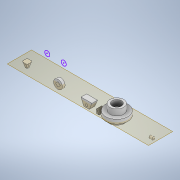
# Autodesk Inventor part: Lab1
Saved by Autodesk Inventor 2021.1 (Build 251245010, 245A)
## iProperties
Created: 2023-09-14
Part Number: Lab1
Material: Типовые
Document SubType Name: Modeling
Designer: Lenovo
Density: 1 g/cm^3
Appearance: По умолчанию
Author: Lenovo
Autodesk Inventor part; units mm, degrees
ref_plane "YZ Plane" through (0, 0, 0) normal (1, 0, 0) x (0, 1, 0)
ref_plane "XY Plane" through (0, 0, 0) normal (0, 0, 1) x (1, 0, 0)
sketch "Эскиз3" plane through (0, 0, 0) normal (0, 0, 1) x (1, 0, 0)
  line L0 (0, 0) -> (10, 0)
  line L1 (10, 0) -> (1.8715, 12.051)
  line L2 (1.8715, 12.051) -> (0, 14.8256)
  line L3 (0, 14.8256) -> (0, 0)
  dimension "d0" = 10
  dimension "d1" = 56
  constraints: 8 end point, 1 horizontal, 1 perpendicular, 1 point on line
  measures "d0" distance of L0.start L0.end
  measures "d1" angle of L1 L0
sketch "Эскиз4" plane through (0, 0, 0) normal (0, 0, 1) x (1, 0, 0)
  line L0 (-46.0484, 0) -> (-26.0484, 0)
  line L1 (-16.0484, 24) -> (-26.0484, 0)
  line L2 (-56.0484, 24) -> (-46.0484, 0)
  circle A0 centre (-36.0484, 8) radius 4
  line L3 (-36.0484, 24) -> (-56.0484, 24)
  line L4 (-36.0484, 24) -> (-16.0484, 24)
  point P0 (0, 0)
  dimension "d2" = 20
  dimension "d8" = 8
  dimension "d10" = 20
  dimension "d11" = 20
  dimension "d12" = 16
  constraints: 10 end point, 2 horizontal, 1 centre point
  measures "d2" distance of L0.start L0.end
  measures "d8" diameter of A0
  measures "d10" distance of L3.start L2.start
  measures "d11" distance of L3.start L1.start
  measures "d12" distance of L3.start A0.centre
sketch "Эскиз5" plane through (0, 0, 0) normal (0, 0, 1) x (1, 0, 0)
  line L0 (60.0217, 0) -> (66.0217, 0)
  line L1 (66.0217, 0) -> (66.0217, 8)
  line L2 (66.0217, 8) -> (74.0217, 8)
  line L3 (74.0217, 8) -> (74.0217, 0)
  line L4 (74.0217, 0) -> (82.0217, 0)
  line L5 (82.0217, 0) -> (82.0217, 12)
  line L6 (82.0217, 12) -> (94.0217, 12)
  line L7 (94.0217, 12) -> (94.0217, 27)
  line L8 (94.0217, 27) -> (79.0217, 27)
  line L9 (79.0217, 27) -> (79.0217, 49)
  line L10 (79.0217, 49) -> (71.0217, 49)
  line L11 (71.0217, 49) -> (71.0217, 29)
  line L12 (71.0217, 29) -> (60.0217, 29)
  line L13 (60.0217, 29) -> (60.0217, 0)
  line L14 (60.0217, 0) -> (54.0217, 0)
  line L15 (54.0217, 15.2415) -> (54.0217, -9.2055)
  point P0 (0, 0)
  dimension "d13" = 6
  dimension "d14" = 8
  dimension "d15" = 8
  dimension "d16" = 8
  dimension "d17" = 8
  dimension "d18" = 12
  dimension "d19" = 12
  dimension "d20" = 15
  dimension "d21" = 15
  dimension "d22" = 22
  dimension "d23" = 8
  dimension "d24" = 20
  dimension "d25" = 11
  dimension "d76" = 6
  constraints: 32 end point, 10 perpendicular, 2 horizontal, 2 point on line, 1 coincident, 1 vertical
  measures "d13" distance of L0.start L0.end
  measures "d14" distance of L0.end L1.end
  measures "d15" distance of L1.end L2.end
  measures "d16" distance of L2.end L3.end
  measures "d17" distance of L3.end L4.end
  measures "d18" distance of L4.end L5.end
  measures "d19" distance of L5.end L6.end
  measures "d20" distance of L6.end L7.end
  measures "d21" distance of L7.end L8.end
  measures "d22" distance of L8.end L9.end
  measures "d23" distance of L9.end L10.end
  measures "d24" distance of L10.end L11.end
  measures "d25" distance of L11.end L12.end
  measures "d76" distance of L0.start L14.end
sketch "Эскиз6" plane through (0, 0, 0) normal (0, 0, 1) x (1, 0, 0)
  circle A0 centre (-150.007, 11.9827) radius 16
  line L0 (-150.007, 20.468) -> (-141.5218, 11.9827)
  line L1 (-158.4923, 11.9827) -> (-150.007, 3.4975)
  line L2 (-150.007, 3.4975) -> (-141.5218, 11.9827)
  line L3 (-141.5218, 11.9827) -> (-150.007, 3.4975)
  line L4 (-158.4923, 11.9827) -> (-150.007, 20.468)
  point P0 (0, 0)
  constraints: 10 end point, 3 perpendicular, 1 centre point
sketch "Эскиз7" plane through (0, 0, 0) normal (0, 0, 1) x (1, 0, 0)
  point P0 (0, 0)
sketch "Эскиз8" plane through (0, 0, 0) normal (0, 0, 1) x (1, 0, 0)
  line L0 (175.9744, 1.9848) -> (175.9744, -0.0152)
  line L1 (175.9744, -0.0152) -> (186.7744, -0.0152)
  line L2 (175.9744, 1.9848) -> (186.7744, 1.9848)
  line L3 (186.7744, 1.9848) -> (186.7744, 1.9848)
  line L4 (187.9744, 3.1848) -> (187.9744, 3.1848)
  line L5 (189.9744, 3.1848) -> (189.9744, 3.1848)
  line L6 (186.7744, -0.0152) -> (186.7744, -0.0152)
  line L7 (186.7744, -0.0152) -> (186.7744, -0.0152)
  line L8 (189.9744, 3.1848) -> (189.9744, 3.4848)
  line L9 (189.9744, 3.4848) -> (187.9744, 3.4848)
  line L10 (187.9744, 3.4848) -> (187.9744, 3.1848)
  line L11 (186.7744, 1.9848) -> (186.7744, 1.9848)
  arc A0 (186.7744, -0.0152) -> (189.9744, 3.1848) centre (186.7744, 3.1848) ccw
  arc A1 (186.7744, 1.9848) -> (187.9744, 3.1848) centre (186.7744, 3.1848) ccw
  line L12 (179.9977, 4.9848) -> (177.4727, 4.9848)
  point P0 (0, 0)
  point P1 (189.9744, -0.0152)
  dimension "d38" = 2
  dimension "d58" = 14
  dimension "d63" = 3.5
  dimension "d64" = 2
  dimension "d67" = 1.2
  dimension "d68" = 3.2
  dimension "d71" = 5
  constraints: 26 end point, 6 perpendicular, 4 horizontal, 4 point on circle, 4 tangent, 2 centre point, 2 point on line, 1 parallel, 1 vertical
  measures "d38" distance of L0.start L0.end
  measures "d58" horizontal distance of L0.end L5.start
  measures "d63" distance of point (189.974, -0.015) L8.end
  measures "d64" distance of L8.end L9.end
  measures "d67" radius of A1
  measures "d68" radius of A0
  measures "d71" distance between parallel lines of L1 L12
extrude "Выдавливание1" add sketch "Эскиз3" along normal blind 20
extrude "Выдавливание2" add sketch "Эскиз6" along normal blind 10
revolve "Вращение1" add sketch "Эскиз5" angle 360 about axis through (54.0217, 15.2415, 0) along (0, -1, 0)
extrude "Выдавливание3" add sketch "Эскиз4" along normal blind 20
revolve "Вращение2" add sketch "Эскиз8" angle 360 about axis through (179.9977, 4.9848, 0) along (-1, 0, 0)
sketch "Эскиз9" plane through (0, 0, 0) normal (0, 1, 0) x (-1, 0, 0)
  circle A0 centre (271.9954, 0) radius 5
  point P0 (0, 0)
  constraints: 1 centre point
ref_plane "РабПлоскость1" through (0, 18, 0) normal (0, 1, 0) x (-1, 0, 0)
sketch "Эскиз10" plane through (0, 18, 0) normal (0, 1, 0) x (-1, 0, 0)
  line L0 (267.1187, 10) -> (277.1187, 10)
  line L1 (282.1187, 5) -> (282.1187, -5)
  line L2 (277.1187, -10) -> (267.1187, -10)
  line L3 (262.1187, -5) -> (262.1187, 5)
  arc A0 (277.1187, -10) -> (282.1187, -5) centre (277.1187, -5) ccw
  arc A1 (262.1187, -5) -> (267.1187, -10) centre (267.1187, -5) ccw
  arc A2 (267.1187, 10) -> (262.1187, 5) centre (267.1187, 5) ccw
  arc A3 (282.1187, 5) -> (277.1187, 10) centre (277.1187, 5) ccw
  point P0 (0, 0)
  dimension "d88" = 5
  constraints: 8 end point, 8 point on circle, 8 tangent, 4 centre point, 3 equal radius, 3 perpendicular
  measures "d88" radius of A0
loft "Лофт1" add profiles "Эскиз10", "Эскиз9"
sketch "Эскиз11" plane through (0, 0, 0) normal (0, 0, 1) x (1, 0, 0)
  circle A0 centre (-199.5369, 79.7312) radius 9
  circle A1 centre (-139.5369, 79.7312) radius 9
  point P0 (0, 0)
  constraints: 2 centre point
